Autodesk Fusion 360 part; units mm, degrees
note: some values were not read from the file. Chosen so that the rebuilt part matches the saved one: which bodies a step acts on.
(part 3 of 3)
equation "d62 = body_W / 2"
equation "d64 = body_H - base_t"
equation "d65 = body_L"
equation "d66 = -side_t"
equation "d68 = -body_W / 2"
equation "d70 = wheel_OD"
equation "d71 = wheel_W"
equation "d73 = body_W / 2"
equation "d75 = wheel_OD"
equation "d76 = -wheel_W"
equation "spinner_gap_W = 70 mm" comment "MOCK layout gap for front spinner - NOT_FOR_MANUFACTURING, confirm with real weapon assembly"
equation "wedge_depth = 50 mm" comment "MOCK front wedge depth (front-to-back) - NOT_FOR_MANUFACTURING placeholder"
equation "d104 = body_H - base_t"
equation "d106 = body_W"
equation "d107 = body_L"
equation "d108 = base_t"
equation "battery_mock_L = 104 mm" comment "CONFIRMED: 3S 2200mAh LiPo typical size (Turnigy/GNB-class, ~500-700 THB Thai retail)"
equation "battery_mock_W = 35 mm" comment "MOCK 3S LiPo envelope width - NOT_FOR_MANUFACTURING"
equation "battery_mock_H = 27 mm" comment "MOCK 3S LiPo envelope height - NOT_FOR_MANUFACTURING"
equation "pcb_t = 1.6 mm" comment "Standard PCB thickness placeholder"
equation "module_mock_L = 25 mm" comment "MOCK small electronics module envelope length (driver/BEC/receiver/disconnect) - NOT_FOR_MANUFACTURING"
equation "module_mock_W = 20 mm" comment "MOCK small electronics module envelope width - NOT_FOR_MANUFACTURING"
equation "module_mock_H = 10 mm" comment "MOCK small electronics module envelope height - NOT_FOR_MANUFACTURING"
equation "tt_gearbox_L = 24 mm" comment "TT motor gearbox length along shaft axis - TYPICAL VALUE, confirm exact supplier datasheet before drilling mount holes"
equation "tt_gearbox_W = 22 mm" comment "TT motor gearbox cross-section width - TYPICAL VALUE, confirm before mount holes"
equation "tt_gearbox_H = 18 mm" comment "TT motor gearbox cross-section height - TYPICAL VALUE, confirm before mount holes"
equation "tt_can_D = 20 mm" comment "TT motor can (motor body) diameter - TYPICAL VALUE"
equation "tt_can_L = 25 mm" comment "TT motor can (motor body) length - TYPICAL VALUE"
equation "tt_shaft_D = 5 mm" comment "TT motor output D-shaft diameter - TYPICAL VALUE, confirm before hub fit"
equation "tt_shaft_L = 10 mm" comment "TT motor output shaft protrusion length - TYPICAL VALUE"
equation "d208 = wheel_OD / 2"
equation "d209 = wheel_OD / 2"
equation "d218 = side_t * 5"
equation "d220 = side_t * 5"
equation "d222 = side_t * 5"
equation "d224 = side_t * 5"
equation "hammer_servo_L = 40.5 mm" comment "CONFIRMED: DS3218MG servo body length (incl. mount tabs), srituhobby.com listing"
equation "hammer_servo_W = 20 mm" comment "CONFIRMED: DS3218MG servo body width"
equation "hammer_servo_H = 40.5 mm" comment "CONFIRMED: DS3218MG servo body height"
equation "hammer_servo_horn_D = 25 mm" comment "MOCK: typical servo horn/spline envelope diameter"
equation "hammer_arm_L = 80 mm" comment "MOCK hammer arm length from pivot to head - NOT_FOR_MANUFACTURING, confirm reach vs chassis geometry"
equation "hammer_head_L = 30 mm" comment "MOCK hammer head length - NOT_FOR_MANUFACTURING"
equation "hammer_head_W = 20 mm" comment "MOCK hammer head width - NOT_FOR_MANUFACTURING"
equation "hammer_head_H = 15 mm" comment "MOCK hammer head height - NOT_FOR_MANUFACTURING"
equation "spinner_motor_D = 27.5 mm" comment "CONFIRMED: A2212 brushless motor can diameter (standard size)"
equation "spinner_motor_L = 30 mm" comment "CONFIRMED: A2212 brushless motor can length (standard size)"
equation "spinner_shaft_D = 4 mm" comment "DECIDED 2026-09-23: 4 mm weapon shaft (separate from the A2212 3.17 mm motor shaft; driven by 1:1 belt) to fit the 624 bearing"
equation "spinner_bearing_OD = 13 mm" comment "DECIDED 2026-09-23: 624 bearing, 4x13x5 mm, bore matches spinner_shaft_D"
equation "spinner_bar_L = 65 mm" comment "MOCK spinner weapon bar length (within spinner_gap_W envelope) - NOT_FOR_MANUFACTURING, needs structural review before fabrication"
equation "spinner_bar_W = 20 mm" comment "MOCK spinner weapon bar width - NOT_FOR_MANUFACTURING"
equation "spinner_bar_T = 6 mm" comment "MOCK spinner weapon bar thickness - NOT_FOR_MANUFACTURING"
equation "esc_L = 45 mm" comment "MOCK typical 30A BLHeli ESC envelope length"
equation "esc_W = 26 mm" comment "MOCK typical 30A ESC envelope width"
equation "esc_H = 8 mm" comment "MOCK typical 30A ESC envelope height"
equation "print_wall_t = 2 mm" comment "3D printed wall thickness placeholder (PETG typical)"
equation "d430 = battery_mock_L"
equation "d431 = battery_mock_W"
equation "d432 = battery_mock_H"
equation "d464 = base_t * 5"
equation "d466 = base_t * 5"
equation "d470 = ground_clearance + base_t"
equation "d473 = ground_clearance + base_t"
equation "d476 = ground_clearance + base_t"
equation "d485 = ground_clearance + base_t"
equation "d486 = -body_W / 2"
equation "d488 = wedge_depth"
equation "d489 = body_H - base_t"
equation "d490 = body_L / 2"
equation "d491 = ( body_W - spinner_gap_W ) / 2"
equation "d495 = ground_clearance + base_t"
equation "d496 = body_W / 2"
equation "d498 = wedge_depth"
equation "d499 = body_H - base_t"
equation "d500 = body_L / 2"
equation "d501 = -( body_W - spinner_gap_W ) / 2"
equation "d505 = ground_clearance + base_t"
equation "m3_clear_d = 3.4 mm" comment "M3 clearance hole dia for CNC/laser-cut aluminum (tight fit)"
equation "m3_clear_d_fdm = 3.6 mm" comment "M3 clearance hole dia for FDM-printed parts (extra 0.2mm for print tolerance)"
equation "standoff_od = 6 mm" comment "M3 corner standoff outer diameter"
equation "standoff_bore_d = 3.2 mm" comment "Standoff through-bore for M3 screw (tap or use nut at one end)"
equation "tt_hole_spacing = 17.5 mm" comment "CONFIRMED: TT motor (all-metal gearbox variant) 2-hole M3 mount spacing, handsontec.com FAM1062 datasheet - verify against exact purchased unit"
equation "a2212_hole_x = 16 mm" comment "CONFIRMED: A2212 brushless motor rear mount hole spacing (short side), widely documented standard"
equation "a2212_hole_y = 19 mm" comment "CONFIRMED: A2212 brushless motor rear mount hole spacing (long side)"
equation "servo_flange_spacing = 49.5 mm" comment "CONFIRMED: standard servo flange mounting hole spacing (DS3218/MG996R-class), servodatabase.com"
equation "mount_plate_t = 3 mm" comment "Motor mounting bracket/plate thickness (aluminum)"
equation "d563 = standoff_od"
equation "d564 = standoff_bore_d"
equation "d565 = standoff_od"
equation "d566 = standoff_bore_d"
equation "d567 = standoff_od"
equation "d568 = standoff_bore_d"
equation "d569 = standoff_od"
equation "d570 = standoff_bore_d"
equation "d578 = side_t * 5"
equation "d580 = side_t * 5"
equation "d588 = base_t * 4"
equation "lip_h = 5 mm" comment "Battery holder side-lip height"
equation "strap_slot_w = 10 mm" comment "Battery strap slot width"
equation "strap_slot_l = 4 mm" comment "Battery strap slot length (thin slit)"
equation "pcb_standoff_h = 3 mm" comment "PCB standoff height (raises board off floor)"
equation "m2_5_clear_d_fdm = 2.9 mm" comment "M2.5 clearance hole for FDM-printed standoffs"
equation "d597 = battery_mock_L"
equation "d598 = battery_mock_W"
equation "d599 = print_wall_t"
equation "d601 = print_wall_t * 5"
equation "d605 = lip_h"
equation "d607 = lip_h"
equation "d639 = base_t * 6"
equation "d641 = base_t * 6"
equation "d643 = base_t * 6"
equation "d645 = base_t * 6"
equation "d657 = side_t * 6"
equation "d659 = side_t * 6"
equation "m2_clear_d = 2.2 mm" comment "M2 clearance hole for small electronics module mounting"
equation "roll_pin_d = 2 mm" comment "Roll pin diameter through shaft+bar - shock-resistant weapon fastening, stronger than friction set-screw alone"
named bodies: "Base_Plate_Al", "Left_Side_Plate_Al", "Right_Side_Plate_Al", "Left_Wheel", "Right_Wheel", "Top_Cover", "Battery_and_Tray", "Front_Wedge_L", "Front_Wedge_R", "Standoff_1", "Standoff_2", "Standoff_3", "Standoff_4", "Battery_Holder", "Batt_Post_1", "Batt_Post_2", "Batt_Post_3", "Batt_Post_4", "Disconnect_Post_1", "Disconnect_Post_2", "Rear_Panel", "Rx_ER6", "Holder_Rx_ER6", "UBEC_5A", "Holder_UBEC_5A", "FingerTech_Switch_Adapter", "FingerTech_Mini_Switch_Envelope", "Lifter_Spatula_62mm", "Lifter_Hinge_Boss", "Lifter_Pivot_Support_L", "Lifter_Pivot_Support_R", "Lifter_Pivot_Pin_6mm", "Repeat_40kg_Servo_MaxEnvelope", "Lifter_Servo_Base_Rail_L", "Lifter_Servo_Base_Rail_R", "Lifter_Aluminium_Horn", "Lifter_Connecting_Rod", "Lifter_Lower_Hard_Stop", "BBB_22mm_Gearmotor_L", "BBB_4mm_Output_Shaft_L", "BBB_Face_Mount_26mm_L", "BBB_Motor_Cradle_L", "Repeat_4mm_Clamp_Hub_L", "BBB_22mm_Gearmotor_R", "BBB_4mm_Output_Shaft_R", "BBB_Face_Mount_26mm_R", "BBB_Motor_Cradle_R", "Repeat_4mm_Clamp_Hub_R", "BBB_Dual_Brushed_ESC_v2_Envelope", "Battery_Clamp_Bar_1", "Battery_Clamp_Bar_2", "Lifter_Servo_Clamp_Bar_L", "Lifter_Servo_Clamp_Post_L_Rear", "Lifter_Servo_Clamp_Post_L_Front", "Lifter_Servo_Clamp_Bar_R", "Lifter_Servo_Clamp_Post_R_Rear", "Lifter_Servo_Clamp_Post_R_Front", "Lifter_Pin_C_Clip_L", "Lifter_Pin_C_Clip_R", "Lifter_Upper_Stop_45deg"
